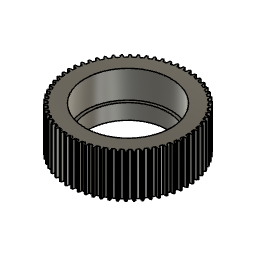
Gear v1 v1 (Autodesk Fusion 360 design; units mm, degrees)
Autodesk Fusion 360 part; units mm, degrees
(part 1 of 2)
sketch "Sketch1" plane through (0, 0, 0) normal (0, 0, 1) x (1, 0, 0)
  circle A0 centre (0, 0) radius 19.5
  dimension "d1" = 39
  constraint coincident A0.centre origin
  measures "d1" diameter of A0
extrude "Extrude1" add sketch "Sketch1" along normal blind 14
sketch "Sketch2" plane through (0, 0, 14) normal (0, 0, 1) x (-1, 0, 0)
  circle A0 centre (0, 0) radius 19.5
  line L0 (0, -18.5) -> (-0.5, -18.5)
  line L1 (-0.5, -18.5) -> (0.5, -18.5)
  line L2 (0, -19.5) -> (-0.75, -19.5)
  line L3 (-0.75, -19.5) -> (0.75, -19.5)
  line L4 (0.75, -19.5) -> (0.5, -18.5)
  line L5 (-0.75, -19.5) -> (-0.5, -18.5)
  dimension "d4" = 1
  dimension "d5" = 0.75
  dimension "d6" = 1.5
  constraint coincident A0 L2.start
  constraint parallel L2 L3
  measures "d4" distance of L2.start L0.start
  measures "d5" distance of L2.start L2.end
  measures "d6" distance of L2.end L3.end
extrude "Extrude2" cut sketch "Sketch2" against normal blind 22.5 contours A0 L0 L1 L4 L5 picked at (-0.2496, -18.8328)
fillet "Fillet2" radius 0.2 2 edges at (-0.5, 18.5, 7) (0.5, 18.5, 7)
fillet "Fillet3" radius 0.1 2 edges at (-0.7464, 19.4857, 7) (0.7464, 19.4857, 7)
pattern_circular "C-Pattern2" count 62 over 360 about axis through (0, 0, 0) along (0, 0, 1) of 7 faces at (-0.7473, 19.447, 9.3333) (-0.6638, 19.155, 9.3333) (-0.5045, 18.5809, 9.3333) (0.1146, 18.5, 9.3333) (0.5045, 18.5809, 9.3333) (0.6638, 19.155, 9.3333) (0.7473, 19.447, 9.3333)
sketch "Sketch3" plane through (0, 0, 14) normal (0, 0, 1) x (-1, 0, 0)
  arc A0 (-1.2404, -19.3807) -> (-1.1473, -19.4662) centre (-1.1414, -19.3664) ccw
  arc A1 (-1.1473, -19.4662) -> (-0.8279, -19.4824) centre (0, 0) ccw
  arc A2 (-0.8279, -19.4824) -> (-0.7267, -19.4068) centre (-0.8237, -19.3825) ccw
  line L0 (-0.7267, -19.4068) -> (-0.5379, -18.6515)
  arc A3 (-0.3438, -18.5) -> (-0.5379, -18.6515) centre (-0.3438, -18.7) ccw
  line L1 (-0.3438, -18.5) -> (0.3438, -18.5)
  arc A4 (0.5379, -18.6515) -> (0.3438, -18.5) centre (0.3438, -18.7) ccw
  line L2 (0.5379, -18.6515) -> (0.7267, -19.4068)
  arc A5 (0.7267, -19.4068) -> (0.8279, -19.4824) centre (0.8237, -19.3825) ccw
  arc A6 (0.8279, -19.4824) -> (1.1473, -19.4662) centre (0, 0) ccw
  arc A7 (1.1473, -19.4662) -> (1.2404, -19.3807) centre (1.1414, -19.3664) ccw
  line L3 (1.2404, -19.3807) -> (1.3518, -18.6102)
  arc A8 (1.5295, -18.4399) -> (1.3518, -18.6102) centre (1.5498, -18.6388) ccw
  line L4 (1.5295, -18.4399) -> (2.2137, -18.3703)
  arc A9 (2.4221, -18.5014) -> (2.2137, -18.3703) centre (2.2339, -18.5693) ccw
  line L5 (2.4221, -18.5014) -> (2.6863, -19.2337)
  arc A10 (2.6863, -19.2337) -> (2.7947, -19.2987) centre (2.7804, -19.1997) ccw
  arc A11 (2.7947, -19.2987) -> (3.1108, -19.2503) centre (0, 0) ccw
  arc A12 (3.1108, -19.2503) -> (3.1947, -19.1558) centre (3.0948, -19.1516) ccw
  line L6 (3.1947, -19.1558) -> (3.2277, -18.378)
  arc A13 (3.3872, -18.1905) -> (3.2277, -18.378) centre (3.4275, -18.3864) ccw
  line L7 (3.3872, -18.1905) -> (4.0608, -18.0521)
  arc A14 (4.2814, -18.1614) -> (4.0608, -18.0521) centre (4.1011, -18.248) ccw
  line L8 (4.2814, -18.1614) -> (4.6184, -18.8632)
  arc A15 (4.6184, -18.8632) -> (4.7328, -18.9169) centre (4.7085, -18.8199) ccw
  arc A16 (4.7328, -18.9169) -> (5.0423, -18.8368) centre (0, 0) ccw
  arc A17 (5.0423, -18.8368) -> (5.1163, -18.7343) centre (5.0165, -18.7402) ccw
  line L9 (5.1163, -18.7343) -> (5.0704, -17.9571)
  arc A18 (5.2101, -17.7545) -> (5.0704, -17.9571) centre (5.27, -17.9453) ccw
  line L10 (5.2101, -17.7545) -> (5.8663, -17.5486)
  arc A19 (6.0968, -17.6351) -> (5.8663, -17.5486) centre (5.9262, -17.7395) ccw
  line L11 (6.0968, -17.6351) -> (6.503, -18.2992)
  arc A20 (6.503, -18.2992) -> (6.6223, -18.3411) centre (6.5883, -18.247) ccw
  arc A21 (6.6223, -18.3411) -> (6.9222, -18.23) centre (0, 0) ccw
  arc A22 (6.9222, -18.23) -> (6.9854, -18.1206) centre (6.8867, -18.1365) ccw
  line L12 (6.9854, -18.1206) -> (6.861, -17.352)
  arc A23 (6.9796, -17.1363) -> (6.861, -17.352) centre (7.0585, -17.3201) ccw
  line L13 (6.9796, -17.1363) -> (7.6116, -16.8651)
  arc A24 (7.8496, -16.9278) -> (7.6116, -16.8651) centre (7.6904, -17.0489) ccw
  line L14 (7.8496, -16.9278) -> (8.321, -17.5474)
  arc A25 (8.321, -17.5474) -> (8.4439, -17.577) centre (8.4006, -17.4869) ccw
  arc A26 (8.4439, -17.577) -> (8.7309, -17.4362) centre (0, 0) ccw
  arc A27 (8.7309, -17.4362) -> (8.7828, -17.3209) centre (8.6862, -17.3468) ccw
  line L15 (8.7828, -17.3209) -> (8.5813, -16.5689)
  arc A28 (8.6774, -16.3423) -> (8.5813, -16.5689) centre (8.7745, -16.5172) ccw
  line L16 (8.6774, -16.3423) -> (9.2787, -16.0085)
  arc A29 (9.5219, -16.0468) -> (9.2787, -16.0085) centre (9.3758, -16.1834) ccw
  line L17 (9.5219, -16.0468) -> (10.0535, -16.6156)
  arc A30 (10.0535, -16.6156) -> (10.1788, -16.6326) centre (10.1266, -16.5473) ccw
  arc A31 (10.1788, -16.6326) -> (10.4501, -16.4634) centre (0, 0) ccw
  arc A32 (10.4501, -16.4634) -> (10.49, -16.3435) centre (10.3965, -16.379) ccw
  line L18 (10.49, -16.3435) -> (10.2135, -15.6157)
  arc A33 (10.2862, -15.3806) -> (10.2135, -15.6157) centre (10.4005, -15.5447) ccw
  line L19 (10.2862, -15.3806) -> (10.8507, -14.9877)
  arc A34 (11.0965, -15.0012) -> (10.8507, -14.9877) centre (10.9649, -15.1518) ccw
  line L20 (11.0965, -15.0012) -> (11.6829, -15.5132)
  arc A35 (11.6829, -15.5132) -> (11.8092, -15.5175) centre (11.7487, -15.4379) ccw
  arc A36 (11.8092, -15.5175) -> (12.0621, -15.3217) centre (0, 0) ccw
  arc A37 (12.0621, -15.3217) -> (12.0896, -15.1984) centre (12.0002, -15.2432) ccw
  line L21 (12.0896, -15.1984) -> (11.741, -14.5023)
  arc A38 (11.7895, -14.261) -> (11.741, -14.5023) centre (11.9198, -14.4127) ccw
  line L22 (11.7895, -14.261) -> (12.3113, -13.8131)
  arc A39 (12.5572, -13.8016) -> (12.3113, -13.8131) centre (12.4416, -13.9648) ccw
  line L23 (12.5572, -13.8016) -> (13.1924, -14.2517)
  arc A40 (13.1924, -14.2517) -> (13.3185, -14.2431) centre (13.2502, -14.1701) ccw
  arc A41 (13.3185, -14.2431) -> (13.5503, -14.0228) centre (0, 0) ccw
  arc A42 (13.5503, -14.0228) -> (13.5652, -13.8973) centre (13.4808, -13.9509) ccw
  line L24 (13.5652, -13.8973) -> (13.1479, -13.2401)
  arc A43 (13.1718, -12.9951) -> (13.1479, -13.2401) centre (13.3167, -13.1329) ccw
  line L25 (13.1718, -12.9951) -> (13.6456, -12.4967)
  arc A44 (13.889, -12.4604) -> (13.6456, -12.4967) centre (13.7905, -12.6345) ccw
  line L26 (13.889, -12.4604) -> (14.5665, -12.8439)
  arc A45 (14.5665, -12.8439) -> (14.6911, -12.8226) centre (14.6158, -12.7569) ccw
  arc A46 (14.6911, -12.8226) -> (14.8994, -12.58) centre (0, 0) ccw
  arc A47 (14.8994, -12.58) -> (14.9016, -12.4536) centre (14.823, -12.5155) ccw
  line L27 (14.9016, -12.4536) -> (14.4199, -11.842)
  arc A48 (14.4189, -11.5959) -> (14.4199, -11.842) centre (14.577, -11.7183) ccw
  line L28 (14.4189, -11.5959) -> (14.8398, -11.0521)
  arc A49 (15.0784, -10.9914) -> (14.8398, -11.0521) centre (14.998, -11.1745) ccw
  line L29 (15.0784, -10.9914) -> (15.7912, -11.3043)
  arc A50 (15.7912, -11.3043) -> (15.913, -11.2706) centre (15.8314, -11.2128) ccw
  arc A51 (15.913, -11.2706) -> (16.0957, -11.0081) centre (0, 0) ccw
  arc A52 (16.0957, -11.0081) -> (16.085, -10.8822) centre (16.0131, -10.9517) ccw
  line L30 (16.085, -10.8822) -> (15.544, -10.3224)
  arc A53 (15.518, -10.0776) -> (15.544, -10.3224) centre (15.6878, -10.1834) ccw
  line L31 (15.518, -10.0776) -> (15.8818, -9.494)
  arc A54 (16.113, -9.4095) -> (15.8818, -9.494) centre (16.0515, -9.5998) ccw
  line L32 (16.113, -9.4095) -> (16.8538, -9.6488)
  arc A55 (16.8538, -9.6488) -> (16.9716, -9.6029) centre (16.8846, -9.5536) ccw
  arc A56 (16.9716, -9.6029) -> (17.1268, -9.3233) centre (0, 0) ccw
  arc A57 (17.1268, -9.3233) -> (17.1034, -9.199) centre (17.0389, -9.2755) ccw
  line L33 (17.1034, -9.199) -> (16.5085, -8.6969)
  arc A58 (16.458, -8.456) -> (16.5085, -8.6969) centre (16.6375, -8.5441) ccw
  line L34 (16.458, -8.456) -> (16.7608, -7.8386)
  arc A59 (16.9823, -7.7311) -> (16.7608, -7.8386) centre (16.9404, -7.9267) ccw
  line L35 (16.9823, -7.7311) -> (17.7435, -7.8942)
  arc A60 (17.7435, -7.8942) -> (17.856, -7.8366) centre (17.7645, -7.7964) ccw
  arc A61 (17.856, -7.8366) -> (17.9821, -7.5428) centre (0, 0) ccw
  arc A62 (17.9821, -7.5428) -> (17.9463, -7.4215) centre (17.8899, -7.5041) ccw
  line L36 (17.9463, -7.4215) -> (17.3037, -6.9822)
  arc A63 (17.229, -6.7476) -> (17.3037, -6.9822) centre (17.4165, -6.817) ccw
  line L37 (17.229, -6.7476) -> (17.4678, -6.1027)
  arc A64 (17.6773, -5.9734) -> (17.4678, -6.1027) centre (17.6554, -6.1722) ccw
  line L38 (17.6773, -5.9734) -> (18.4511, -6.0586)
  arc A65 (18.4511, -6.0586) -> (18.5572, -5.9899) centre (18.4621, -5.9592) ccw
  arc A66 (18.5572, -5.9899) -> (18.653, -5.6848) centre (0, 0) ccw
  arc A67 (18.653, -5.6848) -> (18.6051, -5.5678) centre (18.5573, -5.6557) ccw
  line L39 (18.6051, -5.5678) -> (17.9213, -5.1957)
  arc A68 (17.8232, -4.9699) -> (17.9213, -5.1957) centre (18.0169, -5.0201) ccw
  line L40 (17.8232, -4.9699) -> (17.9956, -4.3042)
  arc A69 (18.1909, -4.1543) -> (17.9956, -4.3042) centre (18.1892, -4.3543) ccw
  line L41 (18.1909, -4.1543) -> (18.9694, -4.1609)
  arc A70 (18.9694, -4.1609) -> (19.068, -4.0818) centre (18.9702, -4.0609) ccw
  arc A71 (19.068, -4.0818) -> (19.1324, -3.7686) centre (0, 0) ccw
  arc A72 (19.1324, -3.7686) -> (19.0729, -3.657) centre (19.0343, -3.7493) ccw
  line L42 (19.0729, -3.657) -> (18.355, -3.356)
  arc A73 (18.2346, -3.1413) -> (18.355, -3.356) centre (18.4323, -3.1716) ccw
  line L43 (18.2346, -3.1413) -> (18.3387, -2.4615)
  arc A74 (18.5179, -2.2927) -> (18.3387, -2.4615) centre (18.5364, -2.4918) ccw
  line L44 (18.5179, -2.2927) -> (19.293, -2.2204)
  arc A75 (19.293, -2.2204) -> (19.3831, -2.1318) centre (19.2837, -2.1208) ccw
  arc A76 (19.3831, -2.1318) -> (19.4155, -1.8137) centre (0, 0) ccw
  arc A77 (19.4155, -1.8137) -> (19.345, -1.7087) centre (19.3159, -1.8044) ccw
  line L45 (19.345, -1.7087) -> (18.6003, -1.4819)
  arc A78 (18.4588, -1.2804) -> (18.6003, -1.4819) centre (18.6586, -1.2905) ccw
  line L46 (18.4588, -1.2804) -> (18.4937, -0.5936)
  arc A79 (18.6548, -0.4075) -> (18.4937, -0.5936) centre (18.6934, -0.6037) ccw
  line L47 (18.6548, -0.4075) -> (19.4187, -0.2572)
  arc A80 (19.4187, -0.2572) -> (19.4993, -0.1599) centre (19.3993, -0.1591) ccw
  arc A81 (19.4993, -0.1599) -> (19.4993, 0.1599) centre (0, 0) ccw
  arc A82 (19.4993, 0.1599) -> (19.4187, 0.2572) centre (19.3993, 0.1591) ccw
  line L48 (19.4187, 0.2572) -> (18.6548, 0.4075)
  arc A83 (18.4937, 0.5936) -> (18.6548, 0.4075) centre (18.6934, 0.6037) ccw
  line L49 (18.4937, 0.5936) -> (18.4588, 1.2804)
  arc A84 (18.6003, 1.4819) -> (18.4588, 1.2804) centre (18.6586, 1.2905) ccw
  line L50 (18.6003, 1.4819) -> (19.345, 1.7087)
  arc A85 (19.345, 1.7087) -> (19.4155, 1.8137) centre (19.3159, 1.8044) ccw
  arc A86 (19.4155, 1.8137) -> (19.3831, 2.1318) centre (0, 0) ccw
  arc A87 (19.3831, 2.1318) -> (19.293, 2.2204) centre (19.2837, 2.1208) ccw
  line L51 (19.293, 2.2204) -> (18.5179, 2.2927)
  arc A88 (18.3387, 2.4615) -> (18.5179, 2.2927) centre (18.5364, 2.4918) ccw
  line L52 (18.3387, 2.4615) -> (18.2346, 3.1413)
  arc A89 (18.355, 3.356) -> (18.2346, 3.1413) centre (18.4323, 3.1716) ccw
  line L53 (18.355, 3.356) -> (19.0729, 3.657)
  arc A90 (19.0729, 3.657) -> (19.1324, 3.7686) centre (19.0343, 3.7493) ccw
  arc A91 (19.1324, 3.7686) -> (19.068, 4.0818) centre (0, 0) ccw
  arc A92 (19.068, 4.0818) -> (18.9694, 4.1609) centre (18.9702, 4.0609) ccw
  line L54 (18.9694, 4.1609) -> (18.1909, 4.1543)
  arc A93 (17.9956, 4.3042) -> (18.1909, 4.1543) centre (18.1892, 4.3543) ccw
  line L55 (17.9956, 4.3042) -> (17.8232, 4.9699)
  arc A94 (17.9213, 5.1957) -> (17.8232, 4.9699) centre (18.0169, 5.0201) ccw
  line L56 (17.9213, 5.1957) -> (18.6051, 5.5678)
  arc A95 (18.6051, 5.5678) -> (18.653, 5.6848) centre (18.5573, 5.6557) ccw
  arc A96 (18.653, 5.6848) -> (18.5572, 5.9899) centre (0, 0) ccw
  arc A97 (18.5572, 5.9899) -> (18.4511, 6.0586) centre (18.4621, 5.9592) ccw
  line L57 (18.4511, 6.0586) -> (17.6773, 5.9734)
  arc A98 (17.4678, 6.1027) -> (17.6773, 5.9734) centre (17.6554, 6.1722) ccw
  line L58 (17.4678, 6.1027) -> (17.229, 6.7476)
  arc A99 (17.3037, 6.9822) -> (17.229, 6.7476) centre (17.4165, 6.817) ccw
  line L59 (17.3037, 6.9822) -> (17.9463, 7.4215)
  arc A100 (17.9463, 7.4215) -> (17.9821, 7.5428) centre (17.8899, 7.5041) ccw
  arc A101 (17.9821, 7.5428) -> (17.856, 7.8366) centre (0, 0) ccw
  arc A102 (17.856, 7.8366) -> (17.7435, 7.8942) centre (17.7645, 7.7964) ccw
  line L60 (17.7435, 7.8942) -> (16.9823, 7.7311)
  arc A103 (16.7608, 7.8386) -> (16.9823, 7.7311) centre (16.9404, 7.9267) ccw
  line L61 (16.7608, 7.8386) -> (16.458, 8.456)
  arc A104 (16.5085, 8.6969) -> (16.458, 8.456) centre (16.6375, 8.5441) ccw
  line L62 (16.5085, 8.6969) -> (17.1034, 9.199)
  arc A105 (17.1034, 9.199) -> (17.1268, 9.3233) centre (17.0389, 9.2755) ccw
  arc A106 (17.1268, 9.3233) -> (16.9716, 9.6029) centre (0, 0) ccw
  arc A107 (16.9716, 9.6029) -> (16.8538, 9.6488) centre (16.8846, 9.5536) ccw
  line L63 (16.8538, 9.6488) -> (16.113, 9.4095)
  arc A108 (15.8818, 9.494) -> (16.113, 9.4095) centre (16.0515, 9.5998) ccw
  line L64 (15.8818, 9.494) -> (15.518, 10.0776)
  arc A109 (15.544, 10.3224) -> (15.518, 10.0776) centre (15.6878, 10.1834) ccw
  line L65 (15.544, 10.3224) -> (16.085, 10.8822)
  arc A110 (16.085, 10.8822) -> (16.0957, 11.0081) centre (16.0131, 10.9517) ccw
  arc A111 (16.0957, 11.0081) -> (15.913, 11.2706) centre (0, 0) ccw
  arc A112 (15.913, 11.2706) -> (15.7912, 11.3043) centre (15.8314, 11.2128) ccw
  line L66 (15.7912, 11.3043) -> (15.0784, 10.9914)
  arc A113 (14.8398, 11.0521) -> (15.0784, 10.9914) centre (14.998, 11.1745) ccw
  line L67 (14.8398, 11.0521) -> (14.4189, 11.5959)
  arc A114 (14.4199, 11.842) -> (14.4189, 11.5959) centre (14.577, 11.7183) ccw
  line L68 (14.4199, 11.842) -> (14.9016, 12.4536)
  arc A115 (14.9016, 12.4536) -> (14.8994, 12.58) centre (14.823, 12.5155) ccw
  arc A116 (14.8994, 12.58) -> (14.6911, 12.8226) centre (0, 0) ccw
  arc A117 (14.6911, 12.8226) -> (14.5665, 12.8439) centre (14.6158, 12.7569) ccw
  line L69 (14.5665, 12.8439) -> (13.889, 12.4604)
  arc A118 (13.6456, 12.4967) -> (13.889, 12.4604) centre (13.7905, 12.6345) ccw
  line L70 (13.6456, 12.4967) -> (13.1718, 12.9951)
  arc A119 (13.1479, 13.2401) -> (13.1718, 12.9951) centre (13.3167, 13.1329) ccw
  line L71 (13.1479, 13.2401) -> (13.5652, 13.8973)
  arc A120 (13.5652, 13.8973) -> (13.5503, 14.0228) centre (13.4808, 13.9509) ccw
  arc A121 (13.5503, 14.0228) -> (13.3185, 14.2431) centre (0, 0) ccw
  arc A122 (13.3185, 14.2431) -> (13.1924, 14.2517) centre (13.2502, 14.1701) ccw
  line L72 (13.1924, 14.2517) -> (12.5572, 13.8016)
  arc A123 (12.3113, 13.8131) -> (12.5572, 13.8016) centre (12.4416, 13.9648) ccw
  line L73 (12.3113, 13.8131) -> (11.7895, 14.261)
  arc A124 (11.741, 14.5023) -> (11.7895, 14.261) centre (11.9198, 14.4127) ccw
  line L74 (11.741, 14.5023) -> (12.0896, 15.1984)
  arc A125 (12.0896, 15.1984) -> (12.0621, 15.3217) centre (12.0002, 15.2432) ccw
  arc A126 (12.0621, 15.3217) -> (11.8092, 15.5175) centre (0, 0) ccw
  arc A127 (11.8092, 15.5175) -> (11.6829, 15.5132) centre (11.7487, 15.4379) ccw
  line L75 (11.6829, 15.5132) -> (11.0965, 15.0012)
  arc A128 (10.8507, 14.9877) -> (11.0965, 15.0012) centre (10.9649, 15.1518) ccw
  line L76 (10.8507, 14.9877) -> (10.2862, 15.3806)
  arc A129 (10.2135, 15.6157) -> (10.2862, 15.3806) centre (10.4005, 15.5447) ccw
  line L77 (10.2135, 15.6157) -> (10.49, 16.3435)
  arc A130 (10.49, 16.3435) -> (10.4501, 16.4634) centre (10.3965, 16.379) ccw
  arc A131 (10.4501, 16.4634) -> (10.1788, 16.6326) centre (0, 0) ccw
  arc A132 (10.1788, 16.6326) -> (10.0535, 16.6156) centre (10.1266, 16.5473) ccw
  line L78 (10.0535, 16.6156) -> (9.5219, 16.0468)
  arc A133 (9.2787, 16.0085) -> (9.5219, 16.0468) centre (9.3758, 16.1834) ccw
  line L79 (9.2787, 16.0085) -> (8.6774, 16.3423)
  arc A134 (8.5813, 16.5689) -> (8.6774, 16.3423) centre (8.7745, 16.5172) ccw
  line L80 (8.5813, 16.5689) -> (8.7828, 17.3209)
  arc A135 (8.7828, 17.3209) -> (8.7309, 17.4362) centre (8.6862, 17.3468) ccw
  arc A136 (8.7309, 17.4362) -> (8.4439, 17.577) centre (0, 0) ccw
  arc A137 (8.4439, 17.577) -> (8.321, 17.5474) centre (8.4006, 17.4869) ccw
  line L81 (8.321, 17.5474) -> (7.8496, 16.9278)
  arc A138 (7.6116, 16.8651) -> (7.8496, 16.9278) centre (7.6904, 17.0489) ccw
  line L82 (7.6116, 16.8651) -> (6.9796, 17.1363)
  arc A139 (6.861, 17.352) -> (6.9796, 17.1363) centre (7.0585, 17.3201) ccw
  line L83 (6.861, 17.352) -> (6.9854, 18.1206)
  arc A140 (6.9854, 18.1206) -> (6.9222, 18.23) centre (6.8867, 18.1365) ccw
  arc A141 (6.9222, 18.23) -> (6.6223, 18.3411) centre (0, 0) ccw
  arc A142 (6.6223, 18.3411) -> (6.503, 18.2992) centre (6.5883, 18.247) ccw
  line L84 (6.503, 18.2992) -> (6.0968, 17.6351)
  arc A143 (5.8663, 17.5486) -> (6.0968, 17.6351) centre (5.9262, 17.7395) ccw
  line L85 (5.8663, 17.5486) -> (5.2101, 17.7545)
  arc A144 (5.0704, 17.9571) -> (5.2101, 17.7545) centre (5.27, 17.9453) ccw
  line L86 (5.0704, 17.9571) -> (5.1163, 18.7343)
  arc A145 (5.1163, 18.7343) -> (5.0423, 18.8368) centre (5.0165, 18.7402) ccw
  arc A146 (5.0423, 18.8368) -> (4.7328, 18.9169) centre (0, 0) ccw
  arc A147 (4.7328, 18.9169) -> (4.6184, 18.8632) centre (4.7085, 18.8199) ccw
  line L87 (4.6184, 18.8632) -> (4.2814, 18.1614)
  arc A148 (4.0608, 18.0521) -> (4.2814, 18.1614) centre (4.1011, 18.248) ccw
  line L88 (4.0608, 18.0521) -> (3.3872, 18.1905)
  arc A149 (3.2277, 18.378) -> (3.3872, 18.1905) centre (3.4275, 18.3864) ccw
  line L89 (3.2277, 18.378) -> (3.1947, 19.1558)
  arc A150 (3.1947, 19.1558) -> (3.1108, 19.2503) centre (3.0948, 19.1516) ccw
  arc A151 (3.1108, 19.2503) -> (2.7947, 19.2987) centre (0, 0) ccw
  arc A152 (2.7947, 19.2987) -> (2.6863, 19.2337) centre (2.7804, 19.1997) ccw
  line L90 (2.6863, 19.2337) -> (2.4221, 18.5014)
  arc A153 (2.2137, 18.3703) -> (2.4221, 18.5014) centre (2.2339, 18.5693) ccw
  line L91 (2.2137, 18.3703) -> (1.5295, 18.4399)
  arc A154 (1.3518, 18.6102) -> (1.5295, 18.4399) centre (1.5498, 18.6388) ccw
  line L92 (1.3518, 18.6102) -> (1.2404, 19.3807)
  arc A155 (1.2404, 19.3807) -> (1.1473, 19.4662) centre (1.1414, 19.3664) ccw
  arc A156 (1.1473, 19.4662) -> (0.8279, 19.4824) centre (0, 0) ccw
  arc A157 (0.8279, 19.4824) -> (0.7267, 19.4068) centre (0.8237, 19.3825) ccw
  line L93 (0.7267, 19.4068) -> (0.5379, 18.6515)
  arc A158 (0.3438, 18.5) -> (0.5379, 18.6515) centre (0.3438, 18.7) ccw
  line L94 (0.3438, 18.5) -> (-0.3438, 18.5)
  arc A159 (-0.5379, 18.6515) -> (-0.3438, 18.5) centre (-0.3438, 18.7) ccw
  line L95 (-0.5379, 18.6515) -> (-0.7267, 19.4068)
  arc A160 (-0.7267, 19.4068) -> (-0.8279, 19.4824) centre (-0.8237, 19.3825) ccw
  arc A161 (-0.8279, 19.4824) -> (-1.1473, 19.4662) centre (0, 0) ccw
  arc A162 (-1.1473, 19.4662) -> (-1.2404, 19.3807) centre (-1.1414, 19.3664) ccw
  line L96 (-1.2404, 19.3807) -> (-1.3518, 18.6102)
  arc A163 (-1.5295, 18.4399) -> (-1.3518, 18.6102) centre (-1.5498, 18.6388) ccw
  line L97 (-1.5295, 18.4399) -> (-2.2137, 18.3703)
  arc A164 (-2.4221, 18.5014) -> (-2.2137, 18.3703) centre (-2.2339, 18.5693) ccw
  line L98 (-2.4221, 18.5014) -> (-2.6863, 19.2337)
  arc A165 (-2.6863, 19.2337) -> (-2.7947, 19.2987) centre (-2.7804, 19.1997) ccw
  arc A166 (-2.7947, 19.2987) -> (-3.1108, 19.2503) centre (0, 0) ccw
  arc A167 (-3.1108, 19.2503) -> (-3.1947, 19.1558) centre (-3.0948, 19.1516) ccw
  line L99 (-3.1947, 19.1558) -> (-3.2277, 18.378)
  arc A168 (-3.3872, 18.1905) -> (-3.2277, 18.378) centre (-3.4275, 18.3864) ccw
  line L100 (-3.3872, 18.1905) -> (-4.0608, 18.0521)
  arc A169 (-4.2814, 18.1614) -> (-4.0608, 18.0521) centre (-4.1011, 18.248) ccw
  line L101 (-4.2814, 18.1614) -> (-4.6184, 18.8632)
  arc A170 (-4.6184, 18.8632) -> (-4.7328, 18.9169) centre (-4.7085, 18.8199) ccw
  arc A171 (-4.7328, 18.9169) -> (-5.0423, 18.8368) centre (0, 0) ccw
  arc A172 (-5.0423, 18.8368) -> (-5.1163, 18.7343) centre (-5.0165, 18.7402) ccw
  line L102 (-5.1163, 18.7343) -> (-5.0704, 17.9571)
  arc A173 (-5.2101, 17.7545) -> (-5.0704, 17.9571) centre (-5.27, 17.9453) ccw
  line L103 (-5.2101, 17.7545) -> (-5.8663, 17.5486)
  arc A174 (-6.0968, 17.6351) -> (-5.8663, 17.5486) centre (-5.9262, 17.7395) ccw
  line L104 (-6.0968, 17.6351) -> (-6.503, 18.2992)
  arc A175 (-6.503, 18.2992) -> (-6.6223, 18.3411) centre (-6.5883, 18.247) ccw
  arc A176 (-6.6223, 18.3411) -> (-6.9222, 18.23) centre (0, 0) ccw
  arc A177 (-6.9222, 18.23) -> (-6.9854, 18.1206) centre (-6.8867, 18.1365) ccw
  line L105 (-6.9854, 18.1206) -> (-6.861, 17.352)
  arc A178 (-6.9796, 17.1363) -> (-6.861, 17.352) centre (-7.0585, 17.3201) ccw
  line L106 (-6.9796, 17.1363) -> (-7.6116, 16.8651)
  arc A179 (-7.8496, 16.9278) -> (-7.6116, 16.8651) centre (-7.6904, 17.0489) ccw
  line L107 (-7.8496, 16.9278) -> (-8.321, 17.5474)
  arc A180 (-8.321, 17.5474) -> (-8.4439, 17.577) centre (-8.4006, 17.4869) ccw
  arc A181 (-8.4439, 17.577) -> (-8.7309, 17.4362) centre (0, 0) ccw
  arc A182 (-8.7309, 17.4362) -> (-8.7828, 17.3209) centre (-8.6862, 17.3468) ccw
  line L108 (-8.7828, 17.3209) -> (-8.5813, 16.5689)
  arc A183 (-8.6774, 16.3423) -> (-8.5813, 16.5689) centre (-8.7745, 16.5172) ccw
  line L109 (-8.6774, 16.3423) -> (-9.2787, 16.0085)
  arc A184 (-9.5219, 16.0468) -> (-9.2787, 16.0085) centre (-9.3758, 16.1834) ccw
  line L110 (-9.5219, 16.0468) -> (-10.0535, 16.6156)
  arc A185 (-10.0535, 16.6156) -> (-10.1788, 16.6326) centre (-10.1266, 16.5473) ccw
  arc A186 (-10.1788, 16.6326) -> (-10.4501, 16.4634) centre (0, 0) ccw
  arc A187 (-10.4501, 16.4634) -> (-10.49, 16.3435) centre (-10.3965, 16.379) ccw
  line L111 (-10.49, 16.3435) -> (-10.2135, 15.6157)
  arc A188 (-10.2862, 15.3806) -> (-10.2135, 15.6157) centre (-10.4005, 15.5447) ccw
  line L112 (-10.2862, 15.3806) -> (-10.8507, 14.9877)
  arc A189 (-11.0965, 15.0012) -> (-10.8507, 14.9877) centre (-10.9649, 15.1518) ccw
  line L113 (-11.0965, 15.0012) -> (-11.6829, 15.5132)
  arc A190 (-11.6829, 15.5132) -> (-11.8092, 15.5175) centre (-11.7487, 15.4379) ccw
  arc A191 (-11.8092, 15.5175) -> (-12.0621, 15.3217) centre (0, 0) ccw
  arc A192 (-12.0621, 15.3217) -> (-12.0896, 15.1984) centre (-12.0002, 15.2432) ccw
  line L114 (-12.0896, 15.1984) -> (-11.741, 14.5023)
  arc A193 (-11.7895, 14.261) -> (-11.741, 14.5023) centre (-11.9198, 14.4127) ccw
  line L115 (-11.7895, 14.261) -> (-12.3113, 13.8131)
  arc A194 (-12.5572, 13.8016) -> (-12.3113, 13.8131) centre (-12.4416, 13.9648) ccw
  line L116 (-12.5572, 13.8016) -> (-13.1924, 14.2517)
  arc A195 (-13.1924, 14.2517) -> (-13.3185, 14.2431) centre (-13.2502, 14.1701) ccw
  arc A196 (-13.3185, 14.2431) -> (-13.5503, 14.0228) centre (0, 0) ccw
  arc A197 (-13.5503, 14.0228) -> (-13.5652, 13.8973) centre (-13.4808, 13.9509) ccw
  line L117 (-13.5652, 13.8973) -> (-13.1479, 13.2401)
  arc A198 (-13.1718, 12.9951) -> (-13.1479, 13.2401) centre (-13.3167, 13.1329) ccw
  line L118 (-13.1718, 12.9951) -> (-13.6456, 12.4967)
  arc A199 (-13.889, 12.4604) -> (-13.6456, 12.4967) centre (-13.7905, 12.6345) ccw
  line L119 (-13.889, 12.4604) -> (-14.5665, 12.8439)
  arc A200 (-14.5665, 12.8439) -> (-14.6911, 12.8226) centre (-14.6158, 12.7569) ccw
  arc A201 (-14.6911, 12.8226) -> (-14.8994, 12.58) centre (0, 0) ccw
  arc A202 (-14.8994, 12.58) -> (-14.9016, 12.4536) centre (-14.823, 12.5155) ccw
  line L120 (-14.9016, 12.4536) -> (-14.4199, 11.842)
  arc A203 (-14.4189, 11.5959) -> (-14.4199, 11.842) centre (-14.577, 11.7183) ccw
  line L121 (-14.4189, 11.5959) -> (-14.8398, 11.0521)
  arc A204 (-15.0784, 10.9914) -> (-14.8398, 11.0521) centre (-14.998, 11.1745) ccw
  line L122 (-15.0784, 10.9914) -> (-15.7912, 11.3043)
  arc A205 (-15.7912, 11.3043) -> (-15.913, 11.2706) centre (-15.8314, 11.2128) ccw
  arc A206 (-15.913, 11.2706) -> (-16.0957, 11.0081) centre (0, 0) ccw
  arc A207 (-16.0957, 11.0081) -> (-16.085, 10.8822) centre (-16.0131, 10.9517) ccw
  line L123 (-16.085, 10.8822) -> (-15.544, 10.3224)
  arc A208 (-15.518, 10.0776) -> (-15.544, 10.3224) centre (-15.6878, 10.1834) ccw
  line L124 (-15.518, 10.0776) -> (-15.8818, 9.494)
  arc A209 (-16.113, 9.4095) -> (-15.8818, 9.494) centre (-16.0515, 9.5998) ccw
  line L125 (-16.113, 9.4095) -> (-16.8538, 9.6488)
  arc A210 (-16.8538, 9.6488) -> (-16.9716, 9.6029) centre (-16.8846, 9.5536) ccw
  arc A211 (-16.9716, 9.6029) -> (-17.1268, 9.3233) centre (0, 0) ccw
  arc A212 (-17.1268, 9.3233) -> (-17.1034, 9.199) centre (-17.0389, 9.2755) ccw
  line L126 (-17.1034, 9.199) -> (-16.5085, 8.6969)
  arc A213 (-16.458, 8.456) -> (-16.5085, 8.6969) centre (-16.6375, 8.5441) ccw
  line L127 (-16.458, 8.456) -> (-16.7608, 7.8386)
  arc A214 (-16.9823, 7.7311) -> (-16.7608, 7.8386) centre (-16.9404, 7.9267) ccw
  line L128 (-16.9823, 7.7311) -> (-17.7435, 7.8942)
  arc A215 (-17.7435, 7.8942) -> (-17.856, 7.8366) centre (-17.7645, 7.7964) ccw
  arc A216 (-17.856, 7.8366) -> (-17.9821, 7.5428) centre (0, 0) ccw
  arc A217 (-17.9821, 7.5428) -> (-17.9463, 7.4215) centre (-17.8899, 7.5041) ccw
  line L129 (-17.9463, 7.4215) -> (-17.3037, 6.9822)
  arc A218 (-17.229, 6.7476) -> (-17.3037, 6.9822) centre (-17.4165, 6.817) ccw
  line L130 (-17.229, 6.7476) -> (-17.4678, 6.1027)
  arc A219 (-17.6773, 5.9734) -> (-17.4678, 6.1027) centre (-17.6554, 6.1722) ccw
  line L131 (-17.6773, 5.9734) -> (-18.4511, 6.0586)
  arc A220 (-18.4511, 6.0586) -> (-18.5572, 5.9899) centre (-18.4621, 5.9592) ccw
  arc A221 (-18.5572, 5.9899) -> (-18.653, 5.6848) centre (0, 0) ccw
  arc A222 (-18.653, 5.6848) -> (-18.6051, 5.5678) centre (-18.5573, 5.6557) ccw
  line L132 (-18.6051, 5.5678) -> (-17.9213, 5.1957)
  arc A223 (-17.8232, 4.9699) -> (-17.9213, 5.1957) centre (-18.0169, 5.0201) ccw
  line L133 (-17.8232, 4.9699) -> (-17.9956, 4.3042)
  arc A224 (-18.1909, 4.1543) -> (-17.9956, 4.3042) centre (-18.1892, 4.3543) ccw
  line L134 (-18.1909, 4.1543) -> (-18.9694, 4.1609)
  arc A225 (-18.9694, 4.1609) -> (-19.068, 4.0818) centre (-18.9702, 4.0609) ccw
  arc A226 (-19.068, 4.0818) -> (-19.1324, 3.7686) centre (0, 0) ccw
  arc A227 (-19.1324, 3.7686) -> (-19.0729, 3.657) centre (-19.0343, 3.7493) ccw
  line L135 (-19.0729, 3.657) -> (-18.355, 3.356)
  arc A228 (-18.2346, 3.1413) -> (-18.355, 3.356) centre (-18.4323, 3.1716) ccw
  line L136 (-18.2346, 3.1413) -> (-18.3387, 2.4615)
  arc A229 (-18.5179, 2.2927) -> (-18.3387, 2.4615) centre (-18.5364, 2.4918) ccw
  line L137 (-18.5179, 2.2927) -> (-19.293, 2.2204)
  arc A230 (-19.293, 2.2204) -> (-19.3831, 2.1318) centre (-19.2837, 2.1208) ccw
  arc A231 (-19.3831, 2.1318) -> (-19.4155, 1.8137) centre (0, 0) ccw
  arc A232 (-19.4155, 1.8137) -> (-19.345, 1.7087) centre (-19.3159, 1.8044) ccw
  line L138 (-19.345, 1.7087) -> (-18.6003, 1.4819)
  arc A233 (-18.4588, 1.2804) -> (-18.6003, 1.4819) centre (-18.6586, 1.2905) ccw
  line L139 (-18.4588, 1.2804) -> (-18.4937, 0.5936)
  arc A234 (-18.6548, 0.4075) -> (-18.4937, 0.5936) centre (-18.6934, 0.6037) ccw
  line L140 (-18.6548, 0.4075) -> (-19.4187, 0.2572)
  arc A235 (-19.4187, 0.2572) -> (-19.4993, 0.1599) centre (-19.3993, 0.1591) ccw
  arc A236 (-19.4993, 0.1599) -> (-19.4993, -0.1599) centre (0, 0) ccw
  arc A237 (-19.4993, -0.1599) -> (-19.4187, -0.2572) centre (-19.3993, -0.1591) ccw
  line L141 (-19.4187, -0.2572) -> (-18.6548, -0.4075)
  arc A238 (-18.4937, -0.5936) -> (-18.6548, -0.4075) centre (-18.6934, -0.6037) ccw
  line L142 (-18.4937, -0.5936) -> (-18.4588, -1.2804)
  arc A239 (-18.6003, -1.4819) -> (-18.4588, -1.2804) centre (-18.6586, -1.2905) ccw
  line L143 (-18.6003, -1.4819) -> (-19.345, -1.7087)
  arc A240 (-19.345, -1.7087) -> (-19.4155, -1.8137) centre (-19.3159, -1.8044) ccw
  arc A241 (-19.4155, -1.8137) -> (-19.3831, -2.1318) centre (0, 0) ccw
  arc A242 (-19.3831, -2.1318) -> (-19.293, -2.2204) centre (-19.2837, -2.1208) ccw
  line L144 (-19.293, -2.2204) -> (-18.5179, -2.2927)
  arc A243 (-18.3387, -2.4615) -> (-18.5179, -2.2927) centre (-18.5364, -2.4918) ccw
  line L145 (-18.3387, -2.4615) -> (-18.2346, -3.1413)
  arc A244 (-18.355, -3.356) -> (-18.2346, -3.1413) centre (-18.4323, -3.1716) ccw
  line L146 (-18.355, -3.356) -> (-19.0729, -3.657)
  arc A245 (-19.0729, -3.657) -> (-19.1324, -3.7686) centre (-19.0343, -3.7493) ccw
  arc A246 (-19.1324, -3.7686) -> (-19.068, -4.0818) centre (0, 0) ccw
  arc A247 (-19.068, -4.0818) -> (-18.9694, -4.1609) centre (-18.9702, -4.0609) ccw
  line L147 (-18.9694, -4.1609) -> (-18.1909, -4.1543)
  arc A248 (-17.9956, -4.3042) -> (-18.1909, -4.1543) centre (-18.1892, -4.3543) ccw
  line L148 (-17.9956, -4.3042) -> (-17.8232, -4.9699)
  arc A249 (-17.9213, -5.1957) -> (-17.8232, -4.9699) centre (-18.0169, -5.0201) ccw
  line L149 (-17.9213, -5.1957) -> (-18.6051, -5.5678)
  arc A250 (-18.6051, -5.5678) -> (-18.653, -5.6848) centre (-18.5573, -5.6557) ccw
  arc A251 (-18.653, -5.6848) -> (-18.5572, -5.9899) centre (0, 0) ccw
  arc A252 (-18.5572, -5.9899) -> (-18.4511, -6.0586) centre (-18.4621, -5.9592) ccw
  line L150 (-18.4511, -6.0586) -> (-17.6773, -5.9734)
  arc A253 (-17.4678, -6.1027) -> (-17.6773, -5.9734) centre (-17.6554, -6.1722) ccw
  line L151 (-17.4678, -6.1027) -> (-17.229, -6.7476)
  arc A254 (-17.3037, -6.9822) -> (-17.229, -6.7476) centre (-17.4165, -6.817) ccw
  line L152 (-17.3037, -6.9822) -> (-17.9463, -7.4215)
  arc A255 (-17.9463, -7.4215) -> (-17.9821, -7.5428) centre (-17.8899, -7.5041) ccw
  arc A256 (-17.9821, -7.5428) -> (-17.856, -7.8366) centre (0, 0) ccw
  arc A257 (-17.856, -7.8366) -> (-17.7435, -7.8942) centre (-17.7645, -7.7964) ccw
  line L153 (-17.7435, -7.8942) -> (-16.9823, -7.7311)
  arc A258 (-16.7608, -7.8386) -> (-16.9823, -7.7311) centre (-16.9404, -7.9267) ccw
  line L154 (-16.7608, -7.8386) -> (-16.458, -8.456)
  arc A259 (-16.5085, -8.6969) -> (-16.458, -8.456) centre (-16.6375, -8.5441) ccw
  line L155 (-16.5085, -8.6969) -> (-17.1034, -9.199)
  arc A260 (-17.1034, -9.199) -> (-17.1268, -9.3233) centre (-17.0389, -9.2755) ccw
  arc A261 (-17.1268, -9.3233) -> (-16.9716, -9.6029) centre (0, 0) ccw
  arc A262 (-16.9716, -9.6029) -> (-16.8538, -9.6488) centre (-16.8846, -9.5536) ccw
  line L156 (-16.8538, -9.6488) -> (-16.113, -9.4095)
  arc A263 (-15.8818, -9.494) -> (-16.113, -9.4095) centre (-16.0515, -9.5998) ccw
  line L157 (-15.8818, -9.494) -> (-15.518, -10.0776)
  arc A264 (-15.544, -10.3224) -> (-15.518, -10.0776) centre (-15.6878, -10.1834) ccw
  line L158 (-15.544, -10.3224) -> (-16.085, -10.8822)
  arc A265 (-16.085, -10.8822) -> (-16.0957, -11.0081) centre (-16.0131, -10.9517) ccw
  arc A266 (-16.0957, -11.0081) -> (-15.913, -11.2706) centre (0, 0) ccw
  arc A267 (-15.913, -11.2706) -> (-15.7912, -11.3043) centre (-15.8314, -11.2128) ccw
  line L159 (-15.7912, -11.3043) -> (-15.0784, -10.9914)
  arc A268 (-14.8398, -11.0521) -> (-15.0784, -10.9914) centre (-14.998, -11.1745) ccw
  line L160 (-14.8398, -11.0521) -> (-14.4189, -11.5959)
  arc A269 (-14.4199, -11.842) -> (-14.4189, -11.5959) centre (-14.577, -11.7183) ccw
  line L161 (-14.4199, -11.842) -> (-14.9016, -12.4536)
  arc A270 (-14.9016, -12.4536) -> (-14.8994, -12.58) centre (-14.823, -12.5155) ccw
  arc A271 (-14.8994, -12.58) -> (-14.6911, -12.8226) centre (0, 0) ccw
  arc A272 (-14.6911, -12.8226) -> (-14.5665, -12.8439) centre (-14.6158, -12.7569) ccw
  line L162 (-14.5665, -12.8439) -> (-13.889, -12.4604)
  arc A273 (-13.6456, -12.4967) -> (-13.889, -12.4604) centre (-13.7905, -12.6345) ccw
  line L163 (-13.6456, -12.4967) -> (-13.1718, -12.9951)
  arc A274 (-13.1479, -13.2401) -> (-13.1718, -12.9951) centre (-13.3167, -13.1329) ccw
  line L164 (-13.1479, -13.2401) -> (-13.5652, -13.8973)
  arc A275 (-13.5652, -13.8973) -> (-13.5503, -14.0228) centre (-13.4808, -13.9509) ccw
  arc A276 (-13.5503, -14.0228) -> (-13.3185, -14.2431) centre (0, 0) ccw
  arc A277 (-13.3185, -14.2431) -> (-13.1924, -14.2517) centre (-13.2502, -14.1701) ccw
  line L165 (-13.1924, -14.2517) -> (-12.5572, -13.8016)
  arc A278 (-12.3113, -13.8131) -> (-12.5572, -13.8016) centre (-12.4416, -13.9648) ccw
  line L166 (-12.3113, -13.8131) -> (-11.7895, -14.261)
  arc A279 (-11.741, -14.5023) -> (-11.7895, -14.261) centre (-11.9198, -14.4127) ccw
  line L167 (-11.741, -14.5023) -> (-12.0896, -15.1984)
  arc A280 (-12.0896, -15.1984) -> (-12.0621, -15.3217) centre (-12.0002, -15.2432) ccw
  arc A281 (-12.0621, -15.3217) -> (-11.8092, -15.5175) centre (0, 0) ccw
  arc A282 (-11.8092, -15.5175) -> (-11.6829, -15.5132) centre (-11.7487, -15.4379) ccw
  line L168 (-11.6829, -15.5132) -> (-11.0965, -15.0012)
  arc A283 (-10.8507, -14.9877) -> (-11.0965, -15.0012) centre (-10.9649, -15.1518) ccw
  line L169 (-10.8507, -14.9877) -> (-10.2862, -15.3806)
  arc A284 (-10.2135, -15.6157) -> (-10.2862, -15.3806) centre (-10.4005, -15.5447) ccw
  line L170 (-10.2135, -15.6157) -> (-10.49, -16.3435)
  arc A285 (-10.49, -16.3435) -> (-10.4501, -16.4634) centre (-10.3965, -16.379) ccw
  arc A286 (-10.4501, -16.4634) -> (-10.1788, -16.6326) centre (0, 0) ccw
  arc A287 (-10.1788, -16.6326) -> (-10.0535, -16.6156) centre (-10.1266, -16.5473) ccw
  line L171 (-10.0535, -16.6156) -> (-9.5219, -16.0468)
  arc A288 (-9.2787, -16.0085) -> (-9.5219, -16.0468) centre (-9.3758, -16.1834) ccw
  line L172 (-9.2787, -16.0085) -> (-8.6774, -16.3423)
  arc A289 (-8.5813, -16.5689) -> (-8.6774, -16.3423) centre (-8.7745, -16.5172) ccw
  line L173 (-8.5813, -16.5689) -> (-8.7828, -17.3209)
  arc A290 (-8.7828, -17.3209) -> (-8.7309, -17.4362) centre (-8.6862, -17.3468) ccw
  arc A291 (-8.7309, -17.4362) -> (-8.4439, -17.577) centre (0, 0) ccw
  arc A292 (-8.4439, -17.577) -> (-8.321, -17.5474) centre (-8.4006, -17.4869) ccw
  line L174 (-8.321, -17.5474) -> (-7.8496, -16.9278)
  arc A293 (-7.6116, -16.8651) -> (-7.8496, -16.9278) centre (-7.6904, -17.0489) ccw
  line L175 (-7.6116, -16.8651) -> (-6.9796, -17.1363)
  arc A294 (-6.861, -17.352) -> (-6.9796, -17.1363) centre (-7.0585, -17.3201) ccw
  line L176 (-6.861, -17.352) -> (-6.9854, -18.1206)
  arc A295 (-6.9854, -18.1206) -> (-6.9222, -18.23) centre (-6.8867, -18.1365) ccw
  arc A296 (-6.9222, -18.23) -> (-6.6223, -18.3411) centre (0, 0) ccw
  arc A297 (-6.6223, -18.3411) -> (-6.503, -18.2992) centre (-6.5883, -18.247) ccw
  line L177 (-6.503, -18.2992) -> (-6.0968, -17.6351)
  arc A298 (-5.8663, -17.5486) -> (-6.0968, -17.6351) centre (-5.9262, -17.7395) ccw
  line L178 (-5.8663, -17.5486) -> (-5.2101, -17.7545)
  arc A299 (-5.0704, -17.9571) -> (-5.2101, -17.7545) centre (-5.27, -17.9453) ccw
  line L179 (-5.0704, -17.9571) -> (-5.1163, -18.7343)
  arc A300 (-5.1163, -18.7343) -> (-5.0423, -18.8368) centre (-5.0165, -18.7402) ccw
  arc A301 (-5.0423, -18.8368) -> (-4.7328, -18.9169) centre (0, 0) ccw
  arc A302 (-4.7328, -18.9169) -> (-4.6184, -18.8632) centre (-4.7085, -18.8199) ccw
  line L180 (-4.6184, -18.8632) -> (-4.2814, -18.1614)
  arc A303 (-4.0608, -18.0521) -> (-4.2814, -18.1614) centre (-4.1011, -18.248) ccw
  line L181 (-4.0608, -18.0521) -> (-3.3872, -18.1905)
  arc A304 (-3.2277, -18.378) -> (-3.3872, -18.1905) centre (-3.4275, -18.3864) ccw
  line L182 (-3.2277, -18.378) -> (-3.1947, -19.1558)
  arc A305 (-3.1947, -19.1558) -> (-3.1108, -19.2503) centre (-3.0948, -19.1516) ccw
  arc A306 (-3.1108, -19.2503) -> (-2.7947, -19.2987) centre (0, 0) ccw
  arc A307 (-2.7947, -19.2987) -> (-2.6863, -19.2337) centre (-2.7804, -19.1997) ccw
  line L183 (-2.6863, -19.2337) -> (-2.4221, -18.5014)
  arc A308 (-2.2137, -18.3703) -> (-2.4221, -18.5014) centre (-2.2339, -18.5693) ccw
  line L184 (-2.2137, -18.3703) -> (-1.5295, -18.4399)
  arc A309 (-1.3518, -18.6102) -> (-1.5295, -18.4399) centre (-1.5498, -18.6388) ccw
  line L185 (-1.3518, -18.6102) -> (-1.2404, -19.3807)
  circle A310 centre (0, 0) radius 13
  dimension "d16" = 26
  constraint coincident A1.centre A6.centre
  measures "d16" diameter of A310
extrude "Extrude3" cut sketch "Sketch3" against normal blind 22 contours A310